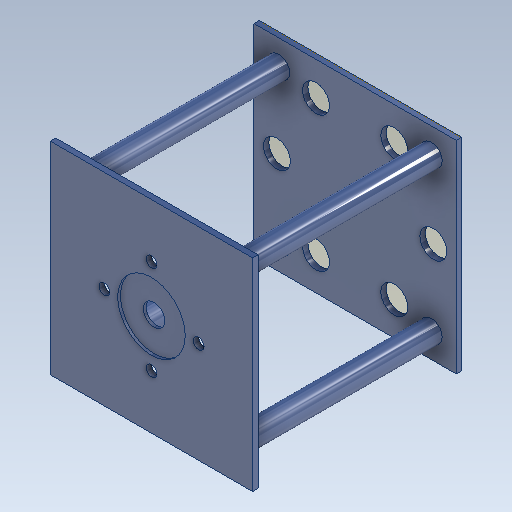
# Autodesk Inventor part: mega troque motor to nmrv-50 flange
Saved by Autodesk Inventor 2020 (Build 240168000, 168)
## iProperties
Created: 2020-08-02
Part Number: mega troque motor to nmrv-50 flange
Material: Generic
Document SubType Name: Modeling
Designer: Vikki
Density: 1 g/cm^3
Appearance: Flaked Satin - Blue
Author: Vikki
Autodesk Inventor part; units mm, degrees
ref_plane "YZ Plane" through (0, 0, 0) normal (1, 0, 0) x (0, 1, 0)
ref_plane "XZ Plane" through (0, 0, 0) normal (0, 1, 0) x (-1, 0, 0)
ref_plane "Work Plane1" through (0, 0, 0) normal (0, 0, 1) x (1, 0, 0)
sketch "Sketch1" plane through (0, 0, 0) normal (0, 0, 1) x (1, 0, 0)
  line L0 (-37.5, -37.5) -> (37.5, -37.5)
  line L1 (37.5, -37.5) -> (37.5, 37.5)
  line L2 (37.5, 37.5) -> (-37.5, 37.5)
  line L3 (-37.5, 37.5) -> (-37.5, -37.5)
  line L4 (-37.5, -37.5) -> (37.5, 37.5) construction
  line L5 (37.5, -37.5) -> (-37.5, 37.5) construction
  circle A0 centre (14.5, 25.1147) radius 5 projected
  circle A1 centre (-14.5, 25.1147) radius 5 projected
  circle A2 centre (-29, 0) radius 5 projected
  circle A3 centre (29, 0) radius 5 projected
  circle A4 centre (14.5, -25.1147) radius 5 projected
  circle A5 centre (-14.5, -25.1147) radius 5 projected
  point P0 (0, 0)
  dimension "d0" = 75
  constraints: 12 end point, 2 midpoint, 2 parallel, 2 perpendicular, 1 horizontal
  measures "d0" distance of L1.end L2.end
extrude "Extrusion1" add sketch "Sketch1" along normal blind 2
sketch "Sketch2" plane through (0, 0, 2) normal (0, 0, 1) x (1, 0, 0)
  circle A0 centre (0, 0) radius 40 construction
  line L0 (28.2843, -28.2843) -> (-28.2843, -28.2843) construction
  line L1 (-28.2843, -28.2843) -> (-28.2843, 28.2843) construction
  line L2 (-28.2843, 28.2843) -> (28.2843, 28.2843) construction
  line L3 (28.2843, 28.2843) -> (28.2843, -28.2843) construction
  line L4 (28.2843, -28.2843) -> (-28.2843, 28.2843) construction
  line L5 (-28.2843, -28.2843) -> (28.2843, 28.2843) construction
  circle A1 centre (-28.2843, 28.2843) radius 4
  circle A2 centre (-28.2843, -28.2843) radius 4
  circle A3 centre (28.2843, -28.2843) radius 4
  circle A4 centre (28.2843, 28.2843) radius 4
  dimension "d3" = 80
  dimension "d4" = 8
  dimension "d7" = 360
  constraints: 12 end point, 4 centre point, 2 coincident, 2 midpoint, 2 parallel, 2 perpendicular, 1 horizontal, 12 other
  measures "d4" diameter of A1
ref_plane "Work Plane2" through (-15.0271, -15.0271, 76.5) normal (0, 0, -1) x (0, 1, 0)
extrude "Extrusion2" add sketch "Sketch2" along normal up to surface (74.5 mm away)
sketch "Sketch3" plane through (28.2843, 28.2843, 76.5) normal (0, 0, 1) x (1, 0, 0)
  circle A0 centre (-45.7843, -28.2843) radius 2 projected
  circle A1 centre (-28.2843, -10.7843) radius 2 projected
  circle A2 centre (-28.2843, -45.7843) radius 2 projected
  circle A3 centre (-10.7843, -28.2843) radius 2 projected
  circle A4 centre (-28.2843, -28.2843) radius 4 projected
  line L0 (-65.7843, 9.2157) -> (-65.7843, -65.7843) projected
  line L1 (9.2157, 9.2157) -> (-65.7843, 9.2157) projected
  line L2 (9.2157, -65.7843) -> (9.2157, 9.2157) projected
  line L3 (-65.7843, -65.7843) -> (9.2157, -65.7843) projected
  point P0 (-28.2843, -28.2843)
extrude "Extrusion3" add sketch "Sketch3" against normal blind 1
sketch "Sketch4" plane through (-37.5, -37.5, 76.5) normal (0, 0, 1) x (1, 0, 0)
  line L0 (0, 75) -> (0, 0) projected
  line L1 (0, 0) -> (75, 0) projected
  line L2 (75, 0) -> (75, 75) projected
  line L3 (75, 75) -> (0, 75) projected
  circle A0 centre (20, 37.5) radius 2 projected
  circle A1 centre (37.5, 55) radius 2 projected
  circle A2 centre (37.5, 20) radius 2 projected
  circle A3 centre (55, 37.5) radius 2 projected
  circle A4 centre (37.5, 37.5) radius 4 projected
  circle A5 centre (37.5, 37.5) radius 12.5 projected
  point P0 (37.5, 37.5)
extrude "Extrusion4" add sketch "Sketch4" along normal blind 1 contours L3 L2 L1 L0
body "Solid1"
